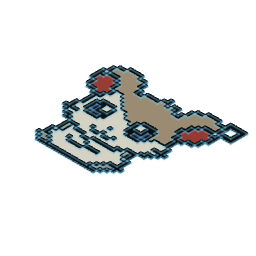
hamster keychain (Autodesk Fusion 360 design; units mm, degrees)
Autodesk Fusion 360 part; units mm, degrees
note: some values were not read from the file. Chosen so that the rebuilt part matches the saved one: which bodies a step acts on.
sketch "hamster" plane through (0, 0, 0) normal (0, 0, 1) x (1, 0, 0)
  line L0 (-33.2218, 24.1948) -> (-33.2218, 28.2088)
  line L1 (-33.2218, 28.2088) -> (-31.192, 28.2088)
  line L2 (-31.192, 28.2088) -> (-31.192, 30.1964)
  line L3 (-31.192, 30.1964) -> (-27.1389, 30.1964)
  line L4 (-27.1389, 30.1964) -> (-27.1389, 32.2747)
  line L5 (-27.1389, 32.2747) -> (-19, 32.2747)
  line L6 (-19, 32.2747) -> (-19, 30.1964)
  line L7 (-19, 30.1964) -> (-15, 30.1964)
  line L8 (-15, 30.1964) -> (-15, 28.2178)
  line L9 (-15, 28.2178) -> (-13, 28.2178)
  line L10 (-13, 28.2178) -> (-13, 24.2275)
  line L11 (-13, 24.2275) -> (-11, 24.2275)
  line L12 (-11, 24.2275) -> (-11, 22.1658)
  line L13 (-11, 22.1658) -> (-8.8499, 22.1658)
  line L14 (-8.8499, 22.1658) -> (-8.8499, 24.2275)
  line L15 (-8.8499, 24.2275) -> (-0.8525, 24.2275)
  line L16 (-0.8525, 24.2275) -> (-0.8525, 26.1894)
  line L17 (-0.8525, 26.1894) -> (1.259, 26.1894)
  line L18 (1.259, 26.1894) -> (1.259, 28.2012)
  line L19 (1.259, 28.2012) -> (3.1711, 28.2012)
  line L20 (3.1711, 28.2012) -> (3.1711, 24.2108)
  line L21 (3.1711, 24.2108) -> (5.266, 24.2108)
  line L22 (5.266, 24.2108) -> (5.266, 26.206)
  line L23 (5.266, 26.206) -> (9.3228, 26.206)
  line L24 (9.3228, 26.206) -> (9.3228, 22.2157)
  line L25 (9.3228, 22.2157) -> (11.3513, 22.2157)
  line L26 (11.3513, 22.2157) -> (11.3513, 24.2108)
  line L27 (11.3513, 24.2108) -> (13.5, 24.2108)
  line L28 (13.5, 24.2108) -> (13.5, 28.2511)
  line L29 (13.5, 28.2511) -> (15.325, 28.2511)
  line L30 (15.325, 28.2511) -> (15.325, 30.2296)
  line L31 (15.325, 30.2296) -> (19.5, 30.2296)
  line L32 (19.5, 30.2296) -> (19.5, 32.2747)
  line L33 (19.5, 32.2747) -> (27.5, 32.2747)
  line L34 (27.5, 32.2747) -> (27.5, 30.2296)
  line L35 (27.5, 30.2296) -> (31.5, 30.2296)
  line L36 (31.5, 30.2296) -> (31.5, 28.2344)
  line L37 (31.5, 28.2344) -> (33.5, 28.2344)
  line L38 (33.5, 28.2344) -> (33.5, 24.2441)
  line L39 (33.5, 24.2441) -> (35.5, 24.2441)
  line L40 (35.5, 24.2441) -> (35.5, 16.1636)
  line L41 (35.5, 16.1636) -> (33.5, 16.1636)
  line L42 (33.5, 16.1636) -> (33.5, 12)
  line L43 (33.5, 12) -> (31.5, 12)
  line L44 (31.5, 12) -> (31.5, 10)
  line L45 (31.5, 10) -> (27.5, 10)
  line L46 (27.5, 10) -> (27.5, 8)
  line L47 (27.5, 8) -> (25.5, 8)
  line L48 (25.5, 8) -> (25.5, 2)
  line L49 (25.5, 2) -> (27.5, 2)
  line L50 (27.5, 2) -> (27.5, -2.1587)
  line L51 (27.5, -2.1587) -> (29.5, -2.1587)
  line L52 (29.5, -2.1587) -> (29.5, -4.1705)
  line L53 (29.5, -4.1705) -> (27.5, -4.1705)
  line L54 (27.5, -4.1705) -> (27.5, -6.1657)
  line L55 (27.5, -6.1657) -> (25.5, -6.1657)
  line L56 (25.5, -6.1657) -> (25.5, -8.1941)
  line L57 (25.5, -8.1941) -> (23.5, -8.1941)
  line L58 (23.5, -8.1941) -> (23.5, -10.2225)
  line L59 (23.5, -10.2225) -> (19.5, -10.2225)
  line L60 (19.5, -10.2225) -> (19.5, -16.3303)
  line L61 (19.5, -16.3303) -> (21.5, -16.3303)
  line L62 (21.5, -16.3303) -> (21.5, -22.5)
  line L63 (21.5, -22.5) -> (23.5, -22.5)
  line L64 (23.5, -22.5) -> (23.5, -24.5)
  line L65 (23.5, -24.5) -> (21.5, -24.5)
  line L66 (21.5, -24.5) -> (21.5, -26.5)
  line L67 (21.5, -26.5) -> (19.5, -26.5)
  line L68 (19.5, -26.5) -> (19.5, -28.5)
  line L69 (19.5, -28.5) -> (17.5, -28.5)
  line L70 (17.5, -28.5) -> (17.5, -30.5)
  line L71 (17.5, -30.5) -> (15.3484, -30.5)
  line L72 (15.3484, -30.5) -> (15.3484, -32.5)
  line L73 (15.3484, -32.5) -> (-19, -32.5)
  line L74 (-19, -32.5) -> (-19, -30.5)
  line L75 (-19, -30.5) -> (-21, -30.5)
  line L76 (-21, -30.5) -> (-21, -28.5)
  line L77 (-21, -28.5) -> (-23, -28.5)
  line L78 (-23, -28.5) -> (-23, -26.5)
  line L79 (-23, -26.5) -> (-21, -26.5)
  line L80 (-21, -26.5) -> (-21, -20.5)
  line L81 (-21, -20.5) -> (-19.2002, -20.5)
  line L82 (-19.2002, -20.5) -> (-19, -20.5)
  line L83 (-19, -20.5) -> (-19, -12.3072)
  line L84 (-19, -12.3072) -> (-23, -12.3072)
  line L85 (-23, -12.3072) -> (-23, -10.2759)
  line L86 (-23, -10.2759) -> (-25, -10.2759)
  line L87 (-25, -10.2759) -> (-25, -8.2446)
  line L88 (-25, -8.2446) -> (-27, -8.2446)
  line L89 (-27, -8.2446) -> (-27, -6.197)
  line L90 (-27, -6.197) -> (-29.1618, -6.197)
  line L91 (-29.1618, -6.197) -> (-29.1618, -4.1819)
  line L92 (-29.1618, -4.1819) -> (-27.163, -4.1819)
  line L93 (-27.163, -4.1819) -> (-27.163, 0)
  line L94 (-27.163, 0) -> (-25.1479, 0)
  line L95 (-25.1479, 0) -> (-25.1479, 8)
  line L96 (-25.1479, 8) -> (-27.1, 8)
  line L97 (-27.1, 8) -> (-27.1, 10)
  line L98 (-27.1, 10) -> (-31.2, 10)
  line L99 (-31.2, 10) -> (-31.2, 12)
  line L100 (-31.2, 12) -> (-33.2, 12)
  line L101 (-33.2, 12) -> (-33.2, 16.1)
  line L102 (-33.2, 16.1) -> (-35.2, 16.1)
  line L103 (-35.2, 16.1) -> (-35.2, 24)
  line L104 (-35.2, 24) -> (-35.2, 24.1948)
  line L105 (-35.2, 24.1948) -> (-33.2218, 24.1948)
  line L106 (-25, -8.2446) -> (-25, -6.2259)
  line L107 (-25, -6.2259) -> (-21, -6.2259)
  line L108 (-21, -6.2259) -> (-21, -4.2404)
  line L109 (-21, -4.2404) -> (-25, -4.2404)
  line L110 (-25, -4.2404) -> (-25, 0)
  line L111 (-25, 0) -> (-23.2, 0)
  line L112 (-23.2, 0) -> (-23.2, 8)
  line L113 (-23.2, 8) -> (-21, 8)
  line L114 (-21, 8) -> (-21, 12)
  line L115 (-21, 12) -> (-19, 12)
  line L116 (-19, 12) -> (-19, 16)
  line L117 (-19, 16) -> (-21, 16)
  line L118 (-21, 16) -> (-21, 12)
  line L119 (-23, 12) -> (-23, 10)
  line L120 (-23, 10) -> (-27, 10)
  line L121 (-27, 10) -> (-27, 12)
  line L122 (-27, 12) -> (-31.2, 12)
  line L123 (-21, 12) -> (-23, 12)
  line L124 (-31.2, 12) -> (-31.2, 16.0945)
  line L125 (-31.2, 16.0945) -> (-33.2, 16.1)
  line L126 (-33.2, 20.1) -> (-31.2, 20.1)
  line L127 (-31.2, 20.1) -> (-31.2, 22.1)
  line L128 (-31.2, 22.1) -> (-33.2, 22.1)
  line L129 (-33.2, 22.1) -> (-33.2218, 24.1948)
  line L130 (-33.2218, 24.1948) -> (-31.2, 24.1948)
  line L131 (-31.2, 24.1948) -> (-31.2, 22.1)
  line L132 (-25.2, 22.1) -> (-25.2, 24.1948)
  line L133 (-25.2, 24.1948) -> (-31.2, 24.1948)
  line L134 (-31.2, 22.1) -> (-23.2, 22.1)
  line L135 (-23.2, 22.1) -> (-23.1, 22.1)
  line L136 (-23.1, 22.1) -> (-23.1, 16.1)
  line L137 (-23.1, 16.1) -> (-23.1, 16)
  line L138 (-23.1, 16) -> (-21, 16)
  line L139 (-21, 20.1301) -> (-25.2, 20.1301)
  line L140 (-25.2, 20.1301) -> (-25.2, 22.1)
  line L141 (-31.2, 24.1948) -> (-31.192, 28.2088)
  line L142 (-31.192, 28.2088) -> (-27.1389, 28.2088)
  line L143 (-27.1389, 28.2088) -> (-27.1389, 30.1964)
  line L144 (-27.1389, 30.1964) -> (-19, 30.1964)
  line L145 (-19, 28.2184) -> (-15, 28.2178)
  line L146 (-19, 28.2184) -> (-19, 30.1964)
  line L147 (-15, 28.2178) -> (-15, 24.2)
  line L148 (-15, 24.2) -> (-13, 24.2275)
  line L149 (-13, 24.2275) -> (-13, 20.1427)
  line L150 (-13, 20.1427) -> (-8.9, 20.1427)
  line L151 (-8.9, 20.1427) -> (-8.8499, 20.1427)
  line L152 (-8.8499, 20.1427) -> (-8.8499, 22.1658)
  line L153 (-8.8499, 22.1658) -> (-0.9, 22.1658)
  line L154 (-0.9, 22.1658) -> (-0.8525, 22.1658)
  line L155 (-0.8525, 22.1658) -> (-0.8525, 24.2275)
  line L156 (-0.8525, 24.2275) -> (3.1711, 24.2108)
  line L157 (3.1711, 22.1648) -> (5.267, 22.1658)
  line L158 (5.267, 22.1658) -> (5.266, 24.2108)
  line L159 (3.1711, 22.1648) -> (3.1711, 24.2108)
  line L160 (5.266, 24.2108) -> (7.3282, 24.2108)
  line L161 (7.3282, 24.2108) -> (7.3282, 22.1648)
  line L162 (7.3282, 22.1648) -> (9.3228, 22.1648)
  line L163 (9.3228, 22.1648) -> (9.3228, 22.2157)
  line L164 (9.3228, 22.1648) -> (9.3228, 20.1507)
  line L165 (9.3228, 20.1507) -> (13.5, 20.1507)
  line L166 (13.5, 20.1507) -> (13.5, 24.2108)
  line L167 (13.5, 24.2108) -> (15.351, 24.2108)
  line L168 (15.351, 24.2108) -> (15.325, 28.2511)
  line L169 (15.325, 28.2511) -> (19.5, 28.2511)
  line L170 (19.5, 28.2511) -> (19.5, 30.2296)
  line L171 (19.5, 30.2296) -> (27.5, 30.2296)
  line L172 (27.5, 30.2296) -> (27.5, 28.2511)
  line L173 (27.5, 28.2511) -> (31.5, 28.2344)
  line L174 (31.5, 28.2344) -> (31.4663, 20.1241)
  line L175 (31.4663, 20.1241) -> (33.5164, 20.1156)
  line L176 (33.5164, 20.1156) -> (33.5, 16.1636)
  line L177 (33.5, 24.2441) -> (25.5, 24.2441)
  line L178 (25.5, 24.2441) -> (25.5, 22.1599)
  line L179 (25.5, 22.1599) -> (33.5, 22.1599)
  line L180 (33.5, 22.1599) -> (33.5, 24.2441)
  line L181 (25.5, 22.1599) -> (25.5, 20.1507)
  line L182 (25.5, 20.1507) -> (21.5, 20.1507)
  line L183 (21.5, 20.1507) -> (21.5, 8)
  line L184 (21.5, 8) -> (23.5, 8)
  line L185 (23.5, 8) -> (23.5, 2)
  line L186 (23.5, 2) -> (25.5, 2)
  line L187 (27.5, 10) -> (27.5, 12)
  line L188 (27.5, 12) -> (31.5, 12)
  line L189 (31.5, 16) -> (31.5, 16.1636)
  line L190 (31.5, 16.1636) -> (33.5, 16.1636)
  line L191 (27.5, 10) -> (23.5, 10)
  line L192 (23.5, 10) -> (23.5, 12)
  line L193 (23.5, 12) -> (19.5, 12)
  line L194 (19.5, 12) -> (19.5, 16.1636)
  line L195 (19.5, 16.1636) -> (23.5, 16.1636)
  line L196 (23.5, 16.1636) -> (23.5, 22.1761)
  line L197 (23.5, 22.1761) -> (25.5, 22.1599)
  line L198 (25.5, 2) -> (25.5, -2.1587)
  line L199 (25.5, -2.1587) -> (21.5, -2.1587)
  line L200 (21.5, -2.1587) -> (21.5, -4.1458)
  line L201 (21.5, -4.1458) -> (25.5, -4.1458)
  line L202 (25.5, -4.1458) -> (25.5, -6.1657)
  line L203 (21.5256, -6.1657) -> (21.5, -8.1584)
  line L204 (21.5, -8.1584) -> (19.5269, -8.133)
  line L205 (19.5269, -8.133) -> (19.5, -10.2225)
  line L206 (19.5, -10.2225) -> (13.4026, -10.2225)
  line L207 (13.4026, -10.2225) -> (13.4026, -14.2426)
  line L208 (13.4026, -14.2426) -> (11.3157, -14.2157)
  line L209 (11.3157, -14.2157) -> (11.3157, -16.3141)
  line L210 (11.3157, -16.3141) -> (-13, -16.3141)
  line L211 (-13, -16.3141) -> (-13, -12.3341)
  line L212 (-13, -12.3341) -> (-19, -12.3072)
  line L213 (-19, -12.3072) -> (-19, -10.2789)
  line L214 (-19, -10.2789) -> (-21, -10.2789)
  line L215 (-21, -10.2789) -> (-21, -8.2073)
  line L216 (-21, -8.2073) -> (-25, -8.2446)
  line L217 (-19, -20.5) -> (-15, -20.5)
  line L218 (-15, -20.5) -> (-15, -14.3241)
  line L219 (-15, -14.3241) -> (-13, -14.3241)
  line L220 (-17.0671, -14.3241) -> (-15, -14.3241)
  line L221 (-17.0671, -14.3241) -> (-17.0671, -22.5)
  line L222 (-17.0671, -22.5) -> (-19, -22.5)
  line L223 (-19, -22.5) -> (-19, -20.5)
  line L224 (-19, -22.5) -> (-19, -24.5)
  line L225 (-19, -24.5) -> (-17, -24.5)
  line L226 (-17, -24.5) -> (-17, -28.5)
  line L227 (-17, -28.5) -> (-13, -28.5)
  line L228 (-13, -28.5) -> (-13, -30.5)
  line L229 (-13, -30.5) -> (9.341, -30.5)
  line L230 (9.341, -30.5) -> (9.341, -28.5)
  line L231 (9.341, -28.5) -> (13.3862, -28.5)
  line L232 (13.3862, -28.5) -> (13.3862, -24.5)
  line L233 (13.3862, -24.5) -> (19.5, -24.5)
  line L234 (19.5, -24.5) -> (19.5, -26.5)
  line L235 (19.5, -26.5) -> (17.5, -26.5)
  line L236 (17.5, -26.5) -> (17.5, -28.5)
  line L237 (15.5, -28.5) -> (17.5, -28.5)
  line L238 (15.3273, -28.5) -> (15.3484, -30.5)
  line L239 (15.3273, -28.5) -> (15.5, -28.5)
  line L240 (15.3484, -30.5) -> (11.3, -30.5)
  line L241 (11.3, -30.5) -> (11.3, -28.5)
  line L242 (11.3, -28.5) -> (11.3, -26.5)
  line L243 (11.3, -26.5) -> (15.3484, -26.5)
  line L244 (15.3484, -26.5) -> (15.3484, -22.4)
  line L245 (15.3484, -22.4) -> (19.5, -22.4)
  line L246 (19.5, -22.4) -> (19.5, -16.3303)
  line L247 (17.4425, -16.3303) -> (17.4242, -18.4319)
  line L248 (17.4242, -18.4319) -> (19.5, -18.4319)
  line L249 (19.5, -16.3303) -> (15.4, -16.3303)
  line L250 (15.4, -16.3303) -> (15.4, -12.2884)
  line L251 (15.4, -12.2884) -> (17.4425, -12.3062)
  line L252 (17.4425, -12.3062) -> (17.4425, -16.3303)
  line L253 (15.4, -12.3062) -> (9.5, -12.3062)
  line L254 (9.5, -12.3062) -> (9.5, -14.3183)
  line L255 (9.5, -14.3183) -> (-2.7785, -14.3183)
  line L256 (-2.7785, -14.3183) -> (-2.7785, -20.3136)
  line L257 (-2.7785, -20.3136) -> (7.2451, -20.3136)
  line L258 (7.2451, -20.3136) -> (7.2451, -22.5)
  line L259 (7.2451, -22.5) -> (-11, -22.5)
  line L260 (-11, -22.5) -> (-11, -20.3136)
  line L261 (-11, -20.3136) -> (-9, -20.3136)
  line L262 (-9, -20.3136) -> (-9, -24.3574)
  line L263 (-9, -24.3574) -> (-0.78, -24.3574)
  line L264 (-0.78, -24.3574) -> (-0.78, -18.3463)
  line L265 (-0.78, -18.3463) -> (-6.8535, -18.3463)
  line L266 (-6.8535, -18.3463) -> (-6.8535, -14.3337)
  line L267 (-6.8535, -14.3337) -> (-13, -14.3241)
  line L268 (5.2466, -10.1963) -> (5.2496, -8.2759)
  line L269 (5.2496, -8.2759) -> (3.2325, -8.2759)
  line L270 (3.2325, -8.2759) -> (3.2263, -12.2417)
  line L271 (3.2263, -12.2417) -> (-0.8113, -12.2417)
  line L272 (-0.8113, -12.2417) -> (-0.805, -8.2759)
  line L273 (-0.805, -8.2759) -> (-2.7941, -8.2759)
  line L274 (-2.7941, -8.2759) -> (-2.8003, -12.2417)
  line L275 (-2.8003, -12.2417) -> (-7, -12.2417)
  line L276 (-7, -12.2417) -> (-6.9938, -8.2759)
  line L277 (-6.9938, -8.2759) -> (-9, -8.2759)
  line L278 (-9, -8.2759) -> (-9, -10.2588)
  line L279 (-9, -10.2588) -> (5.2466, -10.1963)
  line L280 (-0.8581, -6.1369) -> (-0.8662, -4.2943)
  line L281 (-0.8662, -4.2943) -> (-2.8255, -4.2913)
  line L282 (-2.8255, -4.2913) -> (-2.8177, -6.059)
  line L283 (-2.8177, -6.059) -> (-2.8174, -6.1369)
  line L284 (-2.8174, -6.1369) -> (-0.8581, -6.1369)
  line L285 (13.2776, -4.1704) -> (5.2466, -4.2057)
  line L286 (5.2466, -4.2057) -> (5.2466, -2.1219)
  line L287 (5.2466, -2.1219) -> (3.2055, -2.1309)
  line L288 (3.2055, -2.1309) -> (3.17, 5.9635)
  line L289 (3.17, 5.9635) -> (5.2466, 5.9726)
  line L290 (5.2466, 5.9726) -> (5.2466, 7.9801)
  line L291 (5.2466, 7.9801) -> (13.3066, 8.0155)
  line L292 (13.3066, 8.0155) -> (13.3156, 5.968)
  line L293 (13.3156, 5.968) -> (15.323, 5.9768)
  line L294 (15.323, 5.9768) -> (15.3585, -2.1219)
  line L295 (15.3585, -2.1219) -> (7.3015, -2.1219)
  line L296 (7.3015, -2.1219) -> (7.3015, 0)
  line L297 (7.3015, 0) -> (13.5, 0)
  line L298 (13.5, 0) -> (13.5, 4)
  line L299 (13.5, 4) -> (11.33, 3.9905)
  line L300 (11.33, 3.9905) -> (11.33, -2.1219)
  line L301 (13.5, 0) -> (13.5, -4.1366)
  line L302 (13.5, -4.1366) -> (13.5001, -4.1704)
  line L303 (13.5001, -4.1704) -> (13.2776, -4.1704)
  line L304 (5.2466, 5.9726) -> (5.2466, 1.9552)
  line L305 (5.2466, 1.9552) -> (9.3, 1.9552)
  line L306 (9.3, 1.9552) -> (9.2824, 5.9726)
  line L307 (9.2824, 5.9726) -> (5.2466, 5.9726)
  line L308 (3.1878, 1.9163) -> (1.1724, 1.9552)
  line L309 (1.1724, 1.9552) -> (1.1636, 3.9639)
  line L310 (1.1636, 3.9639) -> (-2.8297, 3.9464)
  line L311 (-2.8297, 3.9464) -> (-2.8386, 5.9726)
  line L312 (-2.8386, 5.9726) -> (-4.8688, 5.9726)
  line L313 (-4.8688, 5.9726) -> (-4.8779, 8.0472)
  line L314 (-4.8779, 8.0472) -> (-8.8454, 8.0297)
  line L315 (-8.8454, 8.0297) -> (-8.8544, 10.0737)
  line L316 (-8.8544, 10.0737) -> (-10.91, 10.0647)
  line L317 (-10.91, 10.0647) -> (-10.9184, 11.9734)
  line L318 (-10.9184, 11.9734) -> (-12.974, 11.9644)
  line L319 (-12.974, 11.9644) -> (-12.9832, 14.0631)
  line L320 (-12.9832, 14.0631) -> (-14.9879, 14.0543)
  line L321 (-14.9879, 14.0543) -> (-14.9971, 16.1528)
  line L322 (-14.9971, 16.1528) -> (-19.0028, 16.1352)
  line L323 (-19.0028, 16.1352) -> (-19, 16)
  line L324 (-21, 20.1301) -> (-21, 16)
  line L325 (-33.2, 20.1) -> (-33.2, 16.1)
  line L326 (-11, -4) -> (-11, -2.1232)
  line L327 (-11, -2.1232) -> (-9, -2.1232)
  line L328 (-9, -2.1232) -> (-9, 6)
  line L329 (-9, 6) -> (-11, 6)
  line L330 (-11, 6) -> (-11, 8)
  line L331 (-11, 8) -> (-19, 8)
  line L332 (-19, 8) -> (-19, 6)
  line L333 (-19, 6) -> (-21, 6)
  line L334 (-21, 6) -> (-21, -2)
  line L335 (-21, -2) -> (-13, -2)
  line L336 (-13, -2) -> (-13, 0)
  line L337 (-13, 0) -> (-19, 0)
  line L338 (-19, 0) -> (-19, 4)
  line L339 (-19, 4) -> (-17, 4)
  line L340 (-17, 4) -> (-17, -2)
  line L341 (-19, 0) -> (-19, -4)
  line L342 (-19, -4) -> (-11, -4)
  line L343 (-11, 6) -> (-11, 2)
  line L344 (-11, 2) -> (-15, 2)
  line L345 (-15, 2) -> (-15, 6)
  line L346 (-15, 6) -> (-11, 6)
  line L347 (-19, -30.5) -> (-15, -30.5)
  line L348 (-15, -30.5) -> (-15, -28.5)
  line L349 (-19, -30.5) -> (-19, -28.5)
  line L350 (-19, -28.5) -> (-21, -28.5)
  line L351 (-21, -26.5) -> (-17, -26.5)
  line L352 (-21, -26.5) -> (-21, -28.5)
  line L353 (21.5256, -6.1657) -> (25.5, -6.1657)
  line L354 (15.3407, -0.0234) -> (17.4668, -0.0141)
  line L355 (17.4668, -0.0141) -> (17.4668, 2)
  line L356 (17.4668, 2) -> (23.5, 2)
  line L357 (15.3407, -0.0234) -> (15.3493, -0.0234)
  line L358 (31.5, 12) -> (31.5, 16)
  line L359 (-17, -26.5) -> (-15, -26.5)
  line L360 (-15, -26.5) -> (-15, -28.5)
  line L361 (31.5, 30.2296) -> (31.5, 33.4876)
  line L362 (31.5, 33.4876) -> (41.5, 33.4876)
  line L363 (41.5, 33.4876) -> (41.5, 23.4876)
  line L364 (41.5, 23.4876) -> (35.5, 23.4876)
  line L365 (33.9877, 30.9876) -> (39, 30.9876)
  line L366 (39, 30.9876) -> (39, 26)
  line L367 (39, 26) -> (34, 26)
  line L368 (34, 26) -> (33.9877, 30.9876)
  dimension "d30" = 10
  dimension "d31" = 10
  constraint vertical L0
  constraint perpendicular L0 L1
  constraint perpendicular L1 L2
  constraint perpendicular L2 L3
  constraint perpendicular L3 L4
  constraint perpendicular L2 L5
  constraint perpendicular L5 L6
  constraint perpendicular L6 L7
  constraint perpendicular L7 L8
  constraint perpendicular L8 L9
  constraint perpendicular L9 L10
  constraint perpendicular L8 L11
  constraint perpendicular L11 L12
  constraint perpendicular L12 L13
  constraint perpendicular L13 L14
  constraint perpendicular L14 L15
  constraint perpendicular L13 L16
  constraint perpendicular L16 L17
  constraint perpendicular L17 L18
  constraint perpendicular L18 L19
  constraint perpendicular L19 L20
  constraint perpendicular L20 L21
  constraint perpendicular L19 L22
  constraint perpendicular L22 L23
  constraint perpendicular L19 L24
  constraint perpendicular L24 L25
  constraint perpendicular L25 L26
  constraint perpendicular L26 L27
  constraint perpendicular L27 L28
  constraint perpendicular L28 L29
  constraint perpendicular L29 L30
  constraint perpendicular L30 L31
  constraint perpendicular L31 L32
  constraint perpendicular L30 L33
  constraint perpendicular L33 L34
  constraint perpendicular L34 L35
  constraint perpendicular L33 L36
  constraint perpendicular L36 L37
  constraint perpendicular L33 L38
  constraint perpendicular L36 L39
  constraint perpendicular L39 L40
  constraint perpendicular L40 L41
  constraint perpendicular L41 L42
  constraint perpendicular L40 L43
  constraint perpendicular L41 L44
  constraint perpendicular L44 L45
  constraint perpendicular L41 L46
  constraint perpendicular L46 L47
  constraint perpendicular L47 L48
  constraint perpendicular L46 L49
  constraint perpendicular L47 L50
  constraint perpendicular L50 L51
  constraint perpendicular L47 L52
  constraint perpendicular L52 L53
  constraint perpendicular L47 L54
  constraint perpendicular L52 L55
  constraint perpendicular L55 L56
  constraint perpendicular L56 L57
  constraint perpendicular L55 L58
  constraint perpendicular L58 L59
  constraint perpendicular L59 L60
  constraint perpendicular L60 L61
  constraint perpendicular L61 L62
  constraint perpendicular L62 L63
  constraint perpendicular L63 L64
  constraint perpendicular L64 L65
  constraint perpendicular L63 L66
  constraint perpendicular L66 L67
  constraint perpendicular L67 L68
  constraint perpendicular L68 L69
  constraint perpendicular L67 L70
  constraint perpendicular L68 L71
  constraint perpendicular L71 L72
  constraint perpendicular L68 L73
  constraint perpendicular L71 L74
  constraint perpendicular L68 L75
  constraint perpendicular L71 L76
  constraint perpendicular L68 L77
  constraint perpendicular L71 L78
  constraint perpendicular L68 L79
  constraint perpendicular L79 L80
  constraint perpendicular L68 L81
  constraint parallel L81 L82
  constraint perpendicular L82 L83
  constraint perpendicular L83 L84
  constraint perpendicular L82 L85
  constraint perpendicular L85 L86
  constraint perpendicular L82 L87
  constraint perpendicular L85 L88
  constraint perpendicular L82 L89
  constraint perpendicular L89 L90
  constraint perpendicular L90 L91
  constraint perpendicular L89 L92
  constraint perpendicular L90 L93
  constraint perpendicular L89 L94
  constraint perpendicular L94 L95
  constraint perpendicular L95 L96
  constraint perpendicular L96 L97
  constraint perpendicular L95 L98
  constraint perpendicular L96 L99
  constraint perpendicular L95 L100
  constraint perpendicular L96 L101
  constraint perpendicular L95 L102
  constraint perpendicular L102 L103
  constraint perpendicular L102 L104
  constraint perpendicular L0 L105
  constraint perpendicular L88 L106
  constraint perpendicular L87 L107
  constraint perpendicular L88 L108
  constraint perpendicular L87 L109
  constraint perpendicular L94 L110
  constraint perpendicular L110 L111
  constraint perpendicular L94 L112
  constraint perpendicular L112 L113
  constraint perpendicular L113 L114
  constraint perpendicular L114 L115
  constraint perpendicular L113 L116
  constraint perpendicular L114 L117
  constraint perpendicular L115 L118
  constraint perpendicular L115 L119
  constraint perpendicular L119 L120
  constraint perpendicular L120 L121
  constraint perpendicular L119 L123
  constraint perpendicular L122 L124
  constraint perpendicular L101 L126
  constraint perpendicular L102 L127
  constraint perpendicular L101 L128
  constraint perpendicular L128 L132
  constraint parallel L130 L133
  constraint perpendicular L130 L131
  constraint perpendicular L127 L134
  constraint perpendicular L127 L135
  constraint perpendicular L128 L136
  constraint perpendicular L117 L137
  constraint perpendicular L118 L138
  constraint perpendicular L136 L139
  constraint perpendicular L134 L140
  constraint perpendicular L3 L143
  constraint perpendicular L6 L144
  constraint perpendicular L144 L146
  constraint perpendicular L9 L147
  constraint perpendicular L149 L150
  constraint perpendicular L149 L151
  constraint perpendicular L13 L152
  constraint perpendicular L152 L153
  constraint perpendicular L16 L154
  constraint perpendicular L15 L155
  constraint perpendicular L157 L158
  constraint vertical L159
  constraint perpendicular L21 L161
  constraint perpendicular L24 L162
  constraint perpendicular L25 L163
  constraint perpendicular L162 L164
  constraint perpendicular L164 L165
  constraint perpendicular L27 L166
  constraint perpendicular L166 L167
  constraint perpendicular L30 L169
  constraint perpendicular L31 L170
  constraint perpendicular L34 L171
  constraint perpendicular L171 L172
  constraint perpendicular L173 L174
  constraint perpendicular L174 L175
  constraint perpendicular L175 L176
  constraint perpendicular L38 L177
  constraint perpendicular L39 L178
  constraint perpendicular L38 L179
  constraint perpendicular L177 L180
  constraint perpendicular L179 L181
  constraint perpendicular L181 L182
  constraint perpendicular L182 L183
  constraint perpendicular L183 L184
  constraint perpendicular L182 L185
  constraint perpendicular L48 L186
  constraint perpendicular L45 L187
  constraint perpendicular L44 L188
  constraint perpendicular L43 L189
  constraint parallel L41 L190
  constraint perpendicular L187 L191
  constraint perpendicular L191 L192
  constraint perpendicular L183 L193
  constraint perpendicular L191 L194
  constraint perpendicular L183 L195
  constraint perpendicular L195 L196
  constraint perpendicular L186 L198
  constraint perpendicular L198 L199
  constraint perpendicular L186 L200
  constraint perpendicular L200 L201
  constraint perpendicular L55 L202
  constraint perpendicular L203 L204
  constraint perpendicular L204 L205
  constraint perpendicular L206 L207
  constraint perpendicular L205 L208
  constraint perpendicular L206 L209
  constraint perpendicular L209 L210
  constraint perpendicular L206 L211
  constraint perpendicular L213 L214
  constraint perpendicular L214 L215
  constraint perpendicular L83 L217
  constraint perpendicular L82 L218
  constraint midpoint L211 L219.end
  constraint perpendicular L211 L219
  constraint perpendicular L218 L220
  constraint perpendicular L217 L221
  constraint perpendicular L218 L222
  constraint perpendicular L82 L223
  constraint perpendicular L222 L224
  constraint perpendicular L223 L225
  constraint perpendicular L222 L226
  constraint perpendicular L226 L227
  constraint perpendicular L227 L228
  constraint perpendicular L228 L229
  constraint perpendicular L229 L230
  constraint perpendicular L228 L231
  constraint perpendicular L229 L232
  constraint perpendicular L228 L233
  constraint perpendicular L67 L234
  constraint perpendicular L234 L235
  constraint perpendicular L235 L236
  constraint perpendicular L236 L237
  constraint parallel L237 L239
  constraint perpendicular L72 L240
  constraint coincident L231 L241.end
  constraint perpendicular L231 L241
  constraint perpendicular L231 L242
  constraint perpendicular L241 L243
  constraint perpendicular L231 L244
  constraint perpendicular L241 L245
  constraint coincident L246 L248.end
  constraint perpendicular L246 L248
  constraint perpendicular L60 L249
  constraint perpendicular L249 L250
  constraint perpendicular L247 L251
  constraint perpendicular L249 L252
  constraint coincident L250 L253.start
  constraint perpendicular L207 L253
  constraint perpendicular L61 L254
  constraint perpendicular L207 L255
  constraint perpendicular L61 L256
  constraint perpendicular L207 L257
  constraint perpendicular L61 L258
  constraint perpendicular L207 L259
  constraint perpendicular L61 L260
  constraint perpendicular L207 L261
  constraint perpendicular L61 L262
  constraint perpendicular L262 L263
  constraint perpendicular L257 L264
  constraint perpendicular L262 L265
  constraint perpendicular L210 L266
  constraint perpendicular L267 L268
  constraint perpendicular L211 L269
  constraint perpendicular L267 L270
  constraint perpendicular L211 L271
  constraint perpendicular L267 L272
  constraint perpendicular L211 L273
  constraint perpendicular L267 L274
  constraint perpendicular L211 L275
  constraint perpendicular L267 L276
  constraint perpendicular L211 L277
  constraint perpendicular L279 L280
  constraint perpendicular L268 L281
  constraint perpendicular L279 L282
  constraint perpendicular L279 L283
  constraint horizontal L284
  constraint perpendicular L280 L285
  constraint perpendicular L280 L287
  constraint perpendicular L279 L288
  constraint perpendicular L280 L289
  constraint perpendicular L280 L291
  constraint perpendicular L279 L292
  constraint perpendicular L280 L293
  constraint perpendicular L279 L294
  constraint perpendicular L295 L296
  constraint perpendicular L296 L297
  constraint perpendicular L295 L298
  constraint perpendicular L280 L299
  constraint midpoint L295 L300.end
  constraint perpendicular L295 L300
  constraint perpendicular L285 L302
  constraint perpendicular L301 L303
  constraint perpendicular L290 L305
  constraint perpendicular L289 L306
  constraint perpendicular L304 L307
  constraint midpoint L288 L308.start
  constraint perpendicular L289 L309
  constraint perpendicular L288 L310
  constraint perpendicular L289 L311
  constraint perpendicular L289 L313
  constraint perpendicular L288 L314
  constraint perpendicular L289 L315
  constraint perpendicular L288 L316
  constraint perpendicular L289 L317
  constraint perpendicular L288 L318
  constraint perpendicular L289 L319
  constraint perpendicular L288 L320
  constraint perpendicular L289 L321
  constraint perpendicular L321 L322
  constraint perpendicular L117 L324
  constraint perpendicular L126 L325
  constraint perpendicular L126 L326
  constraint perpendicular L101 L327
  constraint perpendicular L126 L328
  constraint perpendicular L101 L329
  constraint perpendicular L329 L330
  constraint perpendicular L101 L331
  constraint perpendicular L329 L332
  constraint perpendicular L101 L333
  constraint perpendicular L329 L334
  constraint perpendicular L101 L335
  constraint perpendicular L329 L336
  constraint perpendicular L101 L337
  constraint perpendicular L329 L338
  constraint perpendicular L101 L339
  constraint midpoint L335 L340.end
  constraint perpendicular L335 L340
  constraint perpendicular L337 L341
  constraint perpendicular L326 L342
  constraint perpendicular L329 L343
  constraint perpendicular L330 L344
  constraint perpendicular L329 L345
  constraint perpendicular L330 L346
  constraint perpendicular L74 L347
  constraint midpoint L227 L348.end
  constraint perpendicular L227 L348
  constraint perpendicular L347 L349
  constraint perpendicular L76 L350
  constraint midpoint L226 L351.end
  constraint perpendicular L226 L351
  constraint perpendicular L77 L352
  constraint perpendicular L56 L353
  constraint perpendicular L294 L354
  constraint perpendicular L201 L355
  constraint perpendicular L355 L356
  constraint coincident L354 L357.end
  constraint coincident L294 L357.end
  constraint perpendicular L43 L358
  constraint perpendicular L226 L359
  constraint perpendicular L227 L360
  constraint perpendicular L35 L361
  constraint perpendicular L36 L362
  constraint perpendicular L362 L363
  constraint coincident L40 L364.end
  constraint perpendicular L40 L364
  constraint perpendicular L363 L365
  constraint perpendicular L363 L367
  measures "d30" distance of L361.end L362.end
  measures "d31" distance of L362.end L363.end
extrude "Extrude1" add sketch "hamster" along normal blind 1 contours L117 L132 L133 L134 L135 L136 L139 L141 L142 L143 L144 L145 L146 L147 L148 L149 L150 L151 L152 L153 L154 L155 L156 L157 L158 L159 L160 L161 L162 L164 L165 L166 L167 L168 L169 L170 L171 L172 L173 L174 L177 L178 L182 L183 L184 L185 L193 L194 L195 L196 L197 L288 L289 L290 L291 L292 L293 L294 L308 L309 L310 L311 L312 L313 L314 L315 L316 L317 L318 L319 L320 L321 L322 L323 L324 L354 L355 L356 makes body 1
extrude "Extrude2" add sketch "hamster" along normal blind 0.75 contours L46 L47 L48 L183 L184 L185 L186 L191 L192 L193 bodies 1
extrude "Extrude3" add sketch "hamster" along normal blind 0.75 separate body contours L49 L50 L51 L52 L53 L54 L55 L198 L199 L200 L201 L202 makes body 2
extrude "Extrude4" add sketch "hamster" along normal blind 0.75 separate body contours L207 L208 L209 L210 L253 L254 L255 L256 | L60 L206 L207 L249 L250 L251 L252 L253 | L56 L57 L58 L59 L203 L204 L205 L353 | L61 L62 L63 L64 L65 L66 L67 L233 L234 L244 L245 L246 | L42 L43 L189 L190 L358 | L44 L45 L187 L188 makes body 3 at (21.5, -9.5345, 0) makes body 3 at (16.7817, -10.9171, 0) makes body 3 at (20.8333, -20.4101, 0) makes body 3 at (6.0124, -15.6488, 0) makes body 4 at (28.8333, 11.3333, 0) makes body 4 at (32.1667, 14.7758, 0)
extrude "Extrude5" add sketch "hamster" along normal blind 0.75 separate body contours L0 L1 L130 L141 | L131 L132 L133 L134 | L2 L3 L142 L143 | L4 L5 L6 L144 | L7 L8 L145 L146 | L9 L10 L147 L148 | L11 L12 L13 L149 L150 L151 L152 | L14 L15 L153 L154 L155 | L16 L17 L18 L19 L20 L156 | L21 L157 L158 L159 | L22 L23 L24 L160 L161 L162 L163 | L25 L26 L27 L163 L164 L165 L166 | L28 L29 L167 L168 | L30 L31 L169 L170 | L32 L33 L34 L171 | L35 L36 L172 L173 | L37 L38 L174 L177 | L174 L177 L178 L179 | L39 L40 L41 L174 L175 L176 L179 L180 | L181 L182 L196 L197 | L182 L183 L195 L196 | L183 L193 L194 L195 makes body 5 at (12.7838, 22.1924, 0)
extrude "Extrude6" add sketch "hamster" along normal blind 0.75 separate body contours L102 L103 L104 L105 L126 L127 L128 L129 L325 | L134 L135 L136 L139 L140 | L100 L101 L124 L125 | L136 L137 L138 L139 L324 | L88 L89 L90 L91 L92 L93 L94 L95 L96 L97 L98 L99 L106 L107 L108 L109 L110 L111 L112 L113 L114 L119 L120 L121 L122 L123 | L115 L116 L117 L118 | L84 L85 L86 L87 L213 L214 L215 L216 | L83 L211 L212 L217 L219 L220 L221 | L210 L211 L266 L267 | L285 L286 L287 L288 L289 L290 L291 L292 L293 L294 L295 L301 L302 L303 | L268 L269 L270 L279 | L276 L277 L278 L279 | L274 L275 L276 L279 | L272 L273 L274 L279 | L270 L271 L272 L279 | L280 L281 L282 L283 L284 | L326 L327 L328 L329 L330 L331 L332 L333 L334 L335 L341 L342 makes body 7 at (-24.5, 21.4434, 0) makes body 7 at (-22.4, 18.7534, 0) makes body 7 at (-20.3333, 14.6667, 0) makes body 7 at (-24.4493, 5.3333, 0) makes body 7 at (-32.5333, 14.7315, 0) makes body 7 at (-23, -8.9093, 0) makes body 7 at (-34.5333, 20.1316, 0) makes body 7 at (-18.3557, -15.7104, 0) makes body 7 at (-10.9512, -14.9907, 0) makes body 6 at (1.8826, -10.8899, 0) makes body 6 at (3.9029, -9.5591, 0) makes body 6 at (-2.1331, -9.5768, 0) makes body 6 at (-4.1981, -10.9077, 0) makes body 6 at (-8.3323, -9.5949, 0) makes body 9 at (-9.6667, 1.9589, 0) makes body 8 at (-2.1697, -4.9075, 0) makes body 10 at (3.874, 1.9293, 0)
extrude "Extrude7" add sketch "hamster" along normal blind 0.75 separate body contours L80 L81 L82 L223 L224 L225 L226 L351 | L259 L260 L261 L262 | L259 L262 L263 L264 | L257 L258 L259 L264 | L256 L257 L264 L265 | L77 L78 L79 L352 | L210 L256 L265 L266 | L75 L76 L349 L350 | L72 L73 L74 L227 L228 L229 L230 L231 L240 L241 L347 L348 | L70 L71 L237 L238 L239 | L231 L232 L242 L243 | L68 L69 L235 L236 | L232 L233 L243 L244 makes body 11 at (1.8965, -31.8333, 0) makes body 11 at (-20.3333, -29.1667, 0) makes body 11 at (11.9954, -27.1667, 0) makes body 11 at (16.0586, -29.1667, 0) makes body 11 at (-22.3333, -27.1667, 0) makes body 11 at (14.0403, -25.1667, 0) makes body 11 at (18.1667, -27.1667, 0) makes body 11 at (-20.3333, -23.8333, 0) makes body 12 at (-6.26, -23.1191, 0) makes body 12 at (1.895, -21.0424, 0) makes body 12 at (-10.3333, -21.7712, 0) makes body 12 at (-2.1123, -19.0021, 0) makes body 12 at (-4.1368, -17.6689, 0)
extrude "Extrude8" add sketch "hamster" along normal blind 1 separate body contours L217 L221 L222 L223 | L217 L218 L220 L221 | L249 L250 L251 L252 | L246 L247 L248 L249 makes body 13 at (-16.3781, -16.3827, 0) makes body 13 at (-18.3557, -21.1667, 0) makes body 14 at (16.0808, -13.6417, 0) makes body 14 at (18.1222, -17.7314, 0)
extrude "Extrude9" add sketch "hamster" along normal blind 0.5 separate body contours L118 L119 L120 L121 L122 L123 L124 L125 L126 L127 L134 L136 L137 L138 L139 L140 L325 | L226 L227 L347 L348 L349 L350 L351 L352 | L174 L175 L176 L179 L181 L182 L183 L187 L188 L189 L190 L191 L192 L193 L195 L196 L358 | L231 L232 L233 L234 L235 L236 L237 L238 L239 L240 L241 L243 L244 makes body 15 at (-27.1, 14.6982, 0) makes body 16 at (-17, -29.8333, 0) makes body 17 at (27.5, 14.7758, 0) makes body 18 at (17.4495, -25.1667, 0)
extrude "Extrude10" add sketch "hamster" along normal blind 0.5 separate body contours L128 L129 L130 L131 | L106 L107 L108 L109 L110 L111 L112 L113 L114 L115 L116 L186 L198 L199 L200 L201 L202 L203 L204 L205 L206 L207 L210 L211 L212 L213 L214 L215 L216 L253 L254 L255 L256 L266 L267 L285 L286 L287 L288 L294 L295 L301 L302 L303 L308 L309 L310 L311 L312 L313 L314 L315 L316 L317 L318 L319 L320 L321 L322 L323 L353 L354 L355 L356 | L207 L208 L209 L210 L211 L217 L218 L219 L221 L222 L224 L225 L226 L227 L228 L229 L230 L231 L232 L233 L242 L243 L244 L245 L246 L247 L248 L249 L250 L253 L256 L265 L266 L359 L360 | L295 L297 L300 L301 | L304 L305 L306 L307 | L174 L177 L179 L180 | L295 L296 L297 L300 | L297 L298 L299 L300 | L343 L344 L345 L346 | L335 L337 L340 L341 | L335 L336 L337 L340 | L337 L338 L339 L340 makes body 21 at (-4.8851, -0.8227, 0) makes body 21 at (-1.4797, -28.4525, 0) makes body 21 at (12.7767, 0.626, 0) makes body 21 at (-16.3333, -1.3333, 0) makes body 21 at (-13.6667, 4.6667, 0) makes body 19 at (7.943, 3.2943, 0) makes body 20 at (-32.5406, 23.4965, 0) makes body 22 at (32.1527, 22.8546, 0)
extrude "Extrude11" add sketch "hamster" along normal blind 0.75 contours L226 L227 L359 L360 bodies 16 13 18 11 21
combine "Combine1" operation add target body 5 tool bodies 4 7
combine "Combine2" operation add target body 5 tool bodies 12 3
combine "Combine3" operation add target body 5 tool bodies 2
combine "Combine4" operation add target body 10 tool bodies 9 5 makes body 23 at (-9.6667, 1.9589, 0) makes body 24 at (26.1667, 0.6138, 0) makes body 24 at (21.5, -9.5345, 0) makes body 24 at (-10.9512, -14.9907, 0) makes body 24 at (-4.1368, -17.6689, 0) makes body 24 at (6.0124, -15.6488, 0) makes body 24 at (34.8388, 20.1744, 0) makes body 24 at (32.1667, 14.7758, 0) makes body 24 at (-31.8713, 26.8708, 0) makes body 24 at (-34.5333, 20.1316, 0) makes body 24 at (-29.2, 23.4965, 0) makes body 24 at (-24.5, 21.4434, 0.75) makes body 24 at (32.1611, 25.5742, 0) makes body 24 at (29.4861, 23.5494, 0) makes body 24 at (30.1667, 28.905, 0) makes body 24 at (24.1667, 21.4956, 0) makes body 24 at (24.8333, 30.9113, 0) makes body 24 at (22.1667, 18.8217, 0) makes body 24 at (16.7167, 29.5701, 0) makes body 24 at (20.1667, 14.7758, 0) makes body 24 at (14.7253, 25.5576, 0) makes body 24 at (3.8697, 22.8471, 0) makes body 24 at (1.1925, 24.8759, 0) makes body 24 at (-6.1841, 23.5402, 0) makes body 24 at (-10.95, 20.817, 0) makes body 24 at (-14.3333, 25.5484, 0) makes body 24 at (-16.3333, 28.8775, 0) makes body 24 at (-24.426, 31.5819, 0) makes body 24 at (-29.841, 29.5339, 0) makes body 24 at (12.7838, 22.1924, 0) makes body 24 at (28.8333, 11.3333, 0) makes body 24 at (-22.4, 18.7534, 0) makes body 24 at (-20.3333, 14.6667, 0) makes body 24 at (-24.4493, 5.3333, 0) makes body 24 at (-32.5333, 14.7315, 0) makes body 24 at (-23, -8.9093, 0) makes body 24 at (-18.3557, -15.7104, 0) makes body 24 at (-6.26, -23.1191, 0) makes body 24 at (1.895, -21.0424, 0) makes body 24 at (-10.3333, -21.7712, 0) makes body 24 at (-2.1123, -19.0021, 0) makes body 24 at (16.7817, -10.9171, 0) makes body 24 at (20.8333, -20.4101, 0)
combine "Combine5" operation add target body 24 tool bodies 16 14 1 19 10 23 15 17
combine "Combine6" operation add target body 24 tool bodies 18 13 6 8 22 20
extrude "Extrude12" add sketch "hamster" along normal blind 0.75 separate body contours L36 L37 L38 L39 L40 L361 L362 L363 L364 makes body 25
combine "Combine7" operation add target body 24 tool bodies 25
named bodies: "hamster"
